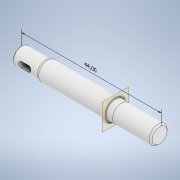
# Autodesk Inventor part: rear shaft v2
Saved by Autodesk Inventor 2022.6 (Build 266554000, 554)
## iProperties
Created: 2024-03-20
Part Number: rear shaft v2
Material: Generic
Document SubType Name: Modeling
Designer: david
Density: 1 g/cm^3
Appearance: Smooth - White
Description: Driving axle
Mass: 1.49261 g
Surface Area: 11.8702 cm^2
Volume: 1.49261 cm^3
Author: david
Autodesk Inventor part; units mm, degrees
ref_plane "YZ Plane" through (0, 0, 0) normal (1, 0, 0) x (0, 1, 0)
ref_plane "XZ Plane" through (0, 0, 0) normal (0, 1, 0) x (-1, 0, 0)
sketch "Sketch1" plane through (0, 0, 0) normal (1, 0, 0) x (0, 1, 0)
  circle A0 centre (0, 0) radius 2.925
  dimension "diameter" = 5.85
  constraints: 1 centre point, 1 coincident
  measures "diameter" diameter of A0
extrude "Shaft" add sketch "Sketch1" along normal mid plane 30
sketch "Sketch2" plane through (0, 0, 0) normal (0, 0, 1) x (1, 0, 0)
  line L0 (-15, -2.925) -> (-15, 2.925) construction
  line L1 (15, -2.925) -> (-15, -2.925) construction
  line L2 (15, 2.925) -> (15, -2.925) construction
  line L3 (-15, 2.925) -> (15, 2.925) construction
  line L4 (-15, -2.925) -> (15, -2.925) projected
  line L5 (-8, -2.925) -> (-8, -2.925)
  line L6 (-15, -2.925) -> (15, -2.925) projected
  line L7 (-13, 0) -> (-9, 0) construction
  line L8 (-12.1, -0.9) -> (-9.9, -0.9)
  line L9 (-9.9, 0.9) -> (-12.1, 0.9)
  arc A0 (-12.1, 0.9) -> (-12.1, -0.9) centre (-12.1, 0) ccw
  arc A1 (-9.9, -0.9) -> (-9.9, 0.9) centre (-9.9, 0) ccw
  point P0 (0, 0)
  point P1 (15, 0)
  point P2 (-11, 0)
  dimension "d17" = 1.8
  dimension "d20" = 2
  dimension "d21" = 1
  dimension "d22" = 7
  constraints: 10 end point, 6 point on circle, 4 tangent, 3 point on line, 2 centre point, 2 midpoint, 1 horizontal, 1 horizontal alignment, 1 parallel, 1 perpendicular, 3 other
  measures "d17" distance between parallel lines of L8 L9
  measures "d20" distance from line of L0 L7.start
  measures "d21" distance from line of L5 L7.end
  measures "d22" distance of L0.start L5.start
extrude "Slot for Differential Gear" cut sketch "Sketch2" along normal through all both and the other way through all
ref_plane "Work Plane1" through (17, 0, 0) normal (1, 0, 0) x (0, 0, -1)
sketch "Sketch3" plane through (17, 0, 0) normal (1, 0, 0) x (0, 0, -1)
  arc A0 (1.6583, -2.5) -> (-1.6583, -2.5) centre (0, 0) ccw construction
  circle A1 centre (0, 0) radius 2.925 construction
  line L0 (-1.6583, -2.5) -> (1.6583, -2.5)
  arc A2 (1.6125, -2.35) -> (-1.6125, -2.35) centre (0, 0) ccw
  line L1 (1.6125, -2.35) -> (-1.6125, -2.35)
  point P0 (-1.5184, -2.5)
  point P1 (1.5184, -2.5)
  dimension "d49" = 3
  dimension "d50" = 2.5
  dimension "wheel_offset" = 0.15
  constraints: 4 end point, 4 point on circle, 2 centre point, 1 coincident, 1 horizontal, 1 other
  measures "d49" radius of A0
  measures "d50" distance from line of L0 A0.centre
  measures "wheel_offset" radial gap between concentric circles of A0 A2
extrude "Wheel Insert Profile" add sketch "Sketch3" along normal blind 12
loft "Loft1" add section 1 edges at (15, -2.925, 0) section 2 edges at (17, -2.35, 0) (17, 2.85, 0)
ref_plane "Work Plane2" through (15, 2.3671, 1.5873) normal (1, 0, 0) x (0, 0, -1)
sketch "Sketch4" plane through (15, 2.3671, 1.5873) normal (1, 0, 0) x (0, 0, -1)
  circle A0 centre (1.5873, -2.3671) radius 3.75
  dimension "d35" = 7.5
  constraints: 1 centre point, 1 coincident
  measures "d35" diameter of A0
extrude "Stopper" add sketch "Sketch4" against normal blind 1
fillet "Fillet1" radius 0.5 2 edges at (15, 0, 3.75) (14, 0, 3.75)
sketch "Sketch8" plane through (-15, 0, 0) normal (-1, 0, 0) x (0, 0, 1)
  circle A0 centre (0, 0) radius 2.925 projected
  circle A1 centre (0, 0) radius 2.7 construction
  circle A2 centre (0, 0) radius 2.65
  dimension "d68" = 5.4
  dimension "d69" = 0.05
  constraints: 2 centre point
  measures "d68" diameter of A1
  measures "d69" radial gap between concentric circles of A1 A2
extrude "Differential Gear Insert Profile" cut sketch "Sketch8" against normal blind 8
fillet "Fillet3" radius 1 1 edges at (-7, -2.925, 0)
chamfer "Chamfer4" distance 0.5 angle 45 2 edges at (-15, 0, -2.65) (29, 2.85, 0)
body "Solid1"
